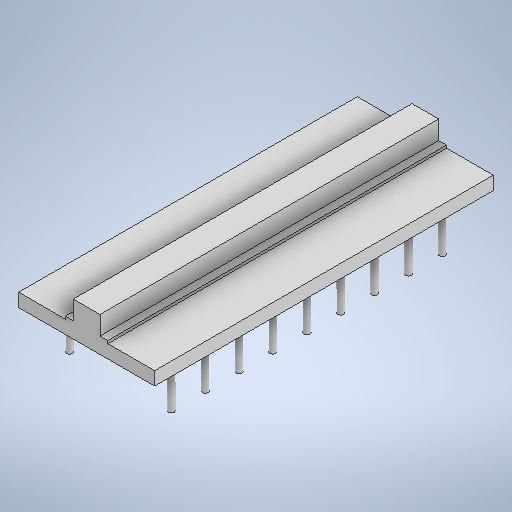
# Autodesk Inventor part: Detector
Saved by Autodesk Inventor 2025 (Build 290162000, 162)
## iProperties
Created: 2025-04-04
Part Number: Detector
Material: Generic
Document SubType Name: Modeling
Designer: nimes
Density: 1 g/cm^3
Appearance: Default
Author: nimes
Autodesk Inventor part; units mm, degrees
ref_plane "YZ Plane" through (0, 0, 0) normal (1, 0, 0) x (0, 1, 0)
ref_plane "XZ Plane" through (0, 0, 0) normal (0, 1, 0) x (-1, 0, 0)
ref_plane "XY Plane" through (0, 0, 0) normal (0, 0, 1) x (1, 0, 0)
sketch "Sketch1" plane through (0, 0, 0) normal (0, 1, 0) x (-1, 0, 0)
  line L0 (0, 0) -> (10.2, 0)
  line L1 (10.2, 0) -> (10.2, -25.4)
  line L2 (10.2, -25.4) -> (0, -25.4)
  line L3 (0, -25.4) -> (0, 0)
  dimension "d0" = 10.2
  dimension "d1" = 25.4
  constraints: 8 end point, 2 parallel, 1 horizontal, 1 perpendicular
  measures "d0" distance of L1.end L2.end
  measures "d1" distance of L0.end L1.end
extrude "Extrusion1" add sketch "Sketch1" along normal blind 1
sketch "Sketch2" plane through (0, 0, 0) normal (0, -1, 0) x (1, 0, 0)
  line L0 (-10.2, -25.4) -> (-10.2, 0) projected
  line L1 (-10.2, 0) -> (-5.1, 0)
  line L2 (-10.2, 0) -> (0, 0) projected
  line L3 (-5.1, 0) -> (-5.1, -25.4)
  line L4 (0, -25.4) -> (-10.2, -25.4) projected
  line L5 (-5.1, -22.7265) -> (-1.29, -22.7265)
  line L6 (-1.29, -22.7265) -> (-1.29, 0)
  line L7 (-1.29, 0) -> (-1.29, -2.54)
  circle A0 centre (-1.29, -2.54) radius 0.5
  line L8 (-1.29, -2.54) -> (-1.29, -5.08)
  line L9 (-1.29, -5.08) -> (-1.29, -7.62)
  line L10 (-1.29, -7.62) -> (-1.29, -10.16)
  line L11 (-1.29, -10.16) -> (-1.29, -12.7)
  line L12 (-1.29, -12.7) -> (-1.29, -15.24)
  line L13 (-1.29, -15.24) -> (-1.29, -17.78)
  line L14 (-1.29, -17.78) -> (-1.29, -20.32)
  line L15 (-1.29, -20.32) -> (-1.29, -22.86)
  circle A1 centre (-1.29, -5.08) radius 0.5
  circle A2 centre (-1.29, -7.62) radius 0.5
  circle A3 centre (-1.29, -10.16) radius 0.5
  circle A4 centre (-1.29, -12.7) radius 0.5
  circle A5 centre (-1.29, -15.24) radius 0.5
  circle A6 centre (-1.29, -17.78) radius 0.5
  circle A7 centre (-1.29, -20.32) radius 0.5
  circle A8 centre (-1.29, -22.86) radius 0.5
  circle A9 centre (-8.91, -2.54) radius 0.5
  circle A10 centre (-8.91, -5.08) radius 0.5
  circle A11 centre (-8.91, -7.62) radius 0.5
  circle A12 centre (-8.91, -10.16) radius 0.5
  circle A13 centre (-8.91, -12.7) radius 0.5
  circle A14 centre (-8.91, -15.24) radius 0.5
  circle A15 centre (-8.91, -17.78) radius 0.5
  circle A16 centre (-8.91, -20.32) radius 0.5
  circle A17 centre (-8.91, -22.86) radius 0.5
  circle A18 centre (-1.29, -22.86) radius 0.225
  circle A19 centre (-1.29, -20.32) radius 0.225
  circle A20 centre (-1.29, -17.78) radius 0.225
  circle A21 centre (-1.29, -15.24) radius 0.225
  circle A22 centre (-1.29, -12.7) radius 0.225
  circle A23 centre (-1.29, -10.16) radius 0.225
  circle A24 centre (-1.29, -7.62) radius 0.225
  circle A25 centre (-1.29, -5.08) radius 0.225
  circle A26 centre (-1.29, -2.54) radius 0.225
  circle A27 centre (-8.91, -22.86) radius 0.225
  circle A28 centre (-8.91, -20.32) radius 0.225
  circle A29 centre (-8.91, -17.78) radius 0.225
  circle A30 centre (-8.91, -15.24) radius 0.225
  circle A31 centre (-8.91, -12.7) radius 0.225
  circle A32 centre (-8.91, -10.16) radius 0.225
  circle A33 centre (-8.91, -7.62) radius 0.225
  circle A34 centre (-8.91, -5.08) radius 0.225
  circle A35 centre (-8.91, -2.54) radius 0.225
  dimension "d4" = 5.1
  dimension "d5" = 90
  dimension "d6" = 3.81
  dimension "d7" = 2.54
  dimension "d8" = 1
  dimension "d9" = 2.54
  dimension "d10" = 2.54
  dimension "d11" = 2.54
  dimension "d12" = 2.54
  dimension "d13" = 2.54
  dimension "d14" = 2.54
  dimension "d15" = 2.54
  dimension "d16" = 2.54
  dimension "d17" = 1
  dimension "d18" = 1
  dimension "d19" = 1
  dimension "d20" = 1
  dimension "d21" = 1
  dimension "d22" = 1
  dimension "d23" = 1
  dimension "d24" = 1
  dimension "d27" = 0.45
  dimension "d28" = 0.45
  dimension "d29" = 0.45
  dimension "d30" = 0.45
  dimension "d31" = 0.45
  dimension "d32" = 0.45
  dimension "d33" = 0.45
  dimension "d34" = 0.45
  dimension "d35" = 0.45
  constraints: 36 centre point, 24 end point, 18 coincident, 18 symmetric about line, 2 horizontal, 2 midpoint, 2 point on line, 30 other
  measures "d4" distance of L0.end L1.end
  measures "d5" angle of L1 L3
  measures "d6" distance of L5.start L5.end
  measures "d7" distance of L7.start L7.end
  measures "d8" diameter of A0
  measures "d9" distance of L8.start L8.end
  measures "d10" distance of L8.end L9.end
  measures "d11" distance of L9.end L10.end
  measures "d12" distance of L10.end L11.end
  measures "d13" distance of L11.end L12.end
  measures "d14" distance of L12.end L13.end
  measures "d15" distance of L13.end L14.end
  measures "d16" distance of L14.end L15.end
  measures "d17" diameter of A1
  measures "d18" diameter of A2
  measures "d19" diameter of A3
  measures "d20" diameter of A4
  measures "d21" diameter of A5
  measures "d22" diameter of A6
  measures "d23" diameter of A7
  measures "d24" diameter of A8
  measures "d27" diameter of A18
  measures "d28" diameter of A19
  measures "d29" diameter of A20
  measures "d30" diameter of A21
  measures "d31" diameter of A22
  measures "d32" diameter of A23
  measures "d33" diameter of A24
  measures "d34" diameter of A25
  measures "d35" diameter of A26
extrude "Extrusion3" add sketch "Sketch2" along normal blind 3.5 contours A18 L6 L5 | L5 L6 A18 | A26 L6 | L6 A26 | A19 L6 | L6 A19 | A25 L6 | L6 A25 | A20 L6 | L6 A20 | A24 L6 | L6 A24 | A21 L6 | L6 A21 | A23 L6 | L6 A23 | A22 L6 | L6 A22 | A27 | A28 | A29 | A30 | A31 | A32 | A33 | A34 | A35
sketch "Sketch3" plane through (0, 0, 0) normal (0, -1, 0) x (1, 0, 0)
  circle A0 centre (-8.91, -22.86) radius 0.225 projected
  circle A1 centre (-8.91, -22.86) radius 0.5
  circle A2 centre (-8.91, -20.32) radius 0.225 projected
  circle A3 centre (-8.91, -20.32) radius 0.5
  circle A4 centre (-8.91, -17.78) radius 0.225 projected
  circle A5 centre (-8.91, -17.78) radius 0.5
  circle A6 centre (-8.91, -15.24) radius 0.225 projected
  circle A7 centre (-8.91, -15.24) radius 0.5
  circle A8 centre (-8.91, -12.7) radius 0.225 projected
  circle A9 centre (-8.91, -12.7) radius 0.5
  circle A10 centre (-8.91, -10.16) radius 0.225 projected
  circle A11 centre (-8.91, -10.16) radius 0.5
  circle A12 centre (-8.91, -7.62) radius 0.225 projected
  circle A13 centre (-8.91, -7.62) radius 0.5
  circle A14 centre (-8.91, -5.08) radius 0.225 projected
  circle A15 centre (-8.91, -5.08) radius 0.5
  circle A16 centre (-8.91, -2.54) radius 0.225 projected
  circle A17 centre (-8.91, -2.54) radius 0.5
  circle A18 centre (-1.29, -22.86) radius 0.225 projected
  circle A19 centre (-1.29, -22.86) radius 0.5
  circle A20 centre (-1.29, -20.32) radius 0.225 projected
  circle A21 centre (-1.29, -20.32) radius 0.5
  circle A22 centre (-1.29, -17.78) radius 0.225 projected
  circle A23 centre (-1.29, -17.78) radius 0.5
  circle A24 centre (-1.29, -15.24) radius 0.225 projected
  circle A25 centre (-1.29, -15.24) radius 0.5
  circle A26 centre (-1.29, -12.7) radius 0.225 projected
  circle A27 centre (-1.29, -12.7) radius 0.5
  circle A28 centre (-1.29, -10.16) radius 0.225 projected
  circle A29 centre (-1.29, -10.16) radius 0.5
  circle A30 centre (-1.29, -7.62) radius 0.225 projected
  circle A31 centre (-1.29, -7.62) radius 0.5
  circle A32 centre (-1.29, -5.08) radius 0.225 projected
  circle A33 centre (-1.29, -5.08) radius 0.5
  circle A34 centre (-1.29, -2.54) radius 0.225 projected
  circle A35 centre (-1.29, -2.54) radius 0.5
  point P0 (0, 0)
  dimension "d38" = 1
  dimension "d39" = 1
  dimension "d40" = 1
  dimension "d41" = 1
  dimension "d42" = 1
  dimension "d43" = 1
  dimension "d44" = 1
  dimension "d45" = 1
  dimension "d46" = 1
  dimension "d47" = 1
  dimension "d48" = 1
  dimension "d49" = 1
  dimension "d50" = 1
  dimension "d51" = 1
  dimension "d52" = 1
  dimension "d53" = 1
  dimension "d54" = 1
  dimension "d55" = 1
  constraints: 18 centre point, 18 coincident
  measures "d38" diameter of A1
  measures "d39" diameter of A3
  measures "d40" diameter of A5
  measures "d41" diameter of A7
  measures "d42" diameter of A9
  measures "d43" diameter of A11
  measures "d44" diameter of A13
  measures "d45" diameter of A15
  measures "d46" diameter of A17
  measures "d47" diameter of A19
  measures "d48" diameter of A21
  measures "d49" diameter of A23
  measures "d50" diameter of A25
  measures "d51" diameter of A27
  measures "d52" diameter of A29
  measures "d53" diameter of A31
  measures "d54" diameter of A33
  measures "d55" diameter of A35
extrude "Extrusion4" add sketch "Sketch3" along normal blind 0.1 contours A0 | A1 | A2 | A3 | A4 | A5 | A6 | A7 | A8 | A9 | A10 | A11 | A12 | A13 | A14 | A15 | A16 | A17 | A18 | A19 | A20 | A21 | A22 | A23 | A24 | A25 | A26 | A27 | A28 | A29 | A30 | A31 | A32 | A33 | A34 | A35
sketch "Sketch5" plane through (0, 1, 0) normal (0, 1, 0) x (1, 0, 0)
  line L0 (0, 0) -> (0, 25.4) projected
  line L1 (0, 0) -> (0, 12.7)
  line L2 (0, 12.7) -> (-5.1, 12.7)
  line L3 (-6.69, 0) -> (-6.69, 25.4)
  line L4 (-6.69, 25.4) -> (-3.51, 25.4)
  line L5 (-3.51, 25.4) -> (-3.51, 0)
  line L6 (-3.51, 0) -> (-6.69, 0)
  line L7 (-6.69, 0) -> (-3.51, 25.4) construction
  line L8 (-6.69, 25.4) -> (-3.51, 0) construction
  dimension "d61" = 12.7
  dimension "d62" = 5.1
  dimension "d63" = 3.18
  constraints: 16 end point, 3 midpoint, 2 parallel, 2 perpendicular
  measures "d61" distance of L0.start L1.end
  measures "d62" distance of L1.end L2.end
  measures "d63" distance of L3.end L4.end
extrude "Extrusion5" add sketch "Sketch5" along normal blind 0.2
sketch "Sketch6" plane through (0, 1.2, 0) normal (0, 1, 0) x (1, 0, 0)
  line L0 (0, 0) -> (0, 12.7)
  line L1 (0, 0) -> (0, 25.4) projected
  line L2 (0, 12.7) -> (-5.1, 12.7)
  line L3 (-6.1, 0) -> (-6.1, 25.4)
  line L4 (-6.1, 25.4) -> (-4.1, 25.4)
  line L5 (-4.1, 25.4) -> (-4.1, 0)
  line L6 (-4.1, 0) -> (-6.1, 0)
  line L7 (-6.1, 0) -> (-4.1, 25.4) construction
  line L8 (-6.1, 25.4) -> (-4.1, 0) construction
  dimension "d66" = 12.7
  dimension "d67" = 5.1
  dimension "d68" = 2
  constraints: 16 end point, 3 midpoint, 3 perpendicular, 2 parallel
  measures "d66" distance of L0.start L0.end
  measures "d67" distance of L0.end L2.end
  measures "d68" distance of L3.end L4.end
extrude "Extrusion6" add sketch "Sketch6" along normal blind 1.4
body "Solid1"
